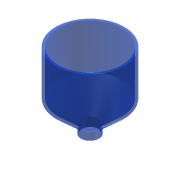
# Autodesk Inventor part: Hopper
Saved by Autodesk Inventor 2014 SP1 (Build 180222100, 222)
## iProperties
Created: 2014-12-12
Part Number: Hopper
Material: Generic
Document SubType Name: Modeling
Designer: AlecShufelt
Density: 1 g/cm^3
Appearance: Clear - Blue
Author: AlecShufelt
Autodesk Inventor part; units mm, degrees
ref_plane "YZ Plane" through (0, 0, 0) normal (1, 0, 0) x (0, 1, 0)
ref_plane "XZ Plane" through (0, 0, 0) normal (0, 1, 0) x (-1, 0, 0)
ref_plane "XY Plane" through (0, 0, 0) normal (0, 0, 1) x (1, 0, 0)
sketch "Sketch1" plane through (0, 0, 0) normal (0, 1, 0) x (-1, 0, 0)
  circle A0 centre (0, 0) radius 10.0965
  dimension "d0" = 20.193
  constraints: 1 centre point, 1 coincident
  measures "d0" diameter of A0
extrude "Extrusion1" add sketch "Sketch1" along normal blind 25.4
sketch "Sketch2" plane through (0, 25.4, 0) normal (0, 1, 0) x (1, 0, 0)
  circle A0 centre (0, 0) radius 10.0965 projected
  circle A1 centre (0, 0) radius 38.1
  dimension "d3" = 76.2
  constraints: 1 centre point, 1 coincident
  measures "d3" diameter of A1
extrude "Extrusion2" add sketch "Sketch2" along normal blind 50.8
loft "Loft1" add section 1 edges at (10.0965, 0, 0) section 2 edges at (-38.1, 25.4, 0)
fillet "Fillet1" radius 3.175 2 edges at (0, 25.4, -38.1) (0, 25.4, 38.1)
sketch "Sketch3" plane through (0, 25.4, 0) normal (0, 1, 0) x (1, 0, 0)
  circle A0 centre (0, 0) radius 10.0965 projected
  circle A1 centre (0, 0) radius 10.0965
  constraints: 1 centre point, 1 coincident, 1 concentric
extrude "Extrusion3" add sketch "Sketch3" along normal blind 50.8
shell "Shell1" thickness 2.54 removed faces 1 at (18.352, 76.2, 0)
sketch "Sketch4" plane through (0, 0, 0) normal (0, -1, 0) x (1, 0, 0)
  circle A0 centre (0, 0) radius 10.0965 projected
  circle A1 centre (0, 0) radius 8.8265
  dimension "d14" = 17.653
  constraints: 1 centre point, 1 coincident
  measures "d14" diameter of A1
extrude "Extrusion4" cut sketch "Sketch4" against normal blind 50.8 contours A1
sketch "Sketch5" plane through (0, 0, 0) normal (0, -1, 0) x (1, 0, 0)
  circle A0 centre (0, 0) radius 8.8265 projected
  circle A1 centre (0, 0) radius 10.0965 projected
  circle A2 centre (0, 0) radius 8.8265
  circle A3 centre (0, 0) radius 10.0965
  constraints: 2 centre point, 2 coincident, 2 concentric
extrude "Extrusion5" add sketch "Sketch5" along normal blind 7.62
body "Solid1"
